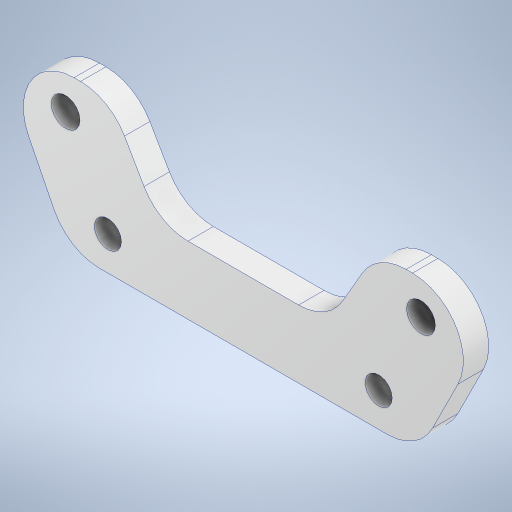
# Autodesk Inventor part: upper_arm
Saved by Autodesk Inventor 2024.1 (Build 281209000, 209)
## iProperties
Created: 2024-02-14
Part Number: upper_arm
Material: アルミニウム 6061
Document SubType Name: Sheet Metal
Designer: hibik
Density: 2.7 g/cm^3
Appearance: アルミニウム - フラット
Sheet Metal Rule: Default
Author: hibik
Autodesk Inventor part; units mm, degrees
ref_plane "YZ Plane" through (0, 0, 0) normal (1, 0, 0) x (0, 1, 0)
ref_plane "XZ Plane" through (0, 0, 0) normal (0, 1, 0) x (-1, 0, 0)
ref_plane "XY Plane" through (0, 0, 0) normal (0, 0, 1) x (1, 0, 0)
sketch "スケッチ2" plane through (0, 0, 0) normal (0, 0, 1) x (1, 0, 0)
  line L0 (0, 0) -> (26, 0)
  line L1 (26, 0) -> (26, 33)
  line L2 (26, 33) -> (0, 33)
  line L3 (0, 33) -> (0, 0)
  line L4 (0, 0) -> (26, 0)
  line L5 (26, 0) -> (26, 24)
  line L6 (26, 24) -> (0, 24) construction
  line L7 (0, 24) -> (0, 0)
  circle A0 centre (13, 24) radius 13
  circle A1 centre (13, 24) radius 6.25
  line L8 (26, 0) -> (0, 0)
  line L9 (0, 0) -> (0, -4)
  line L10 (0, -4) -> (26, -4)
  line L11 (26, -4) -> (26, 0)
  circle A2 centre (21, -2) radius 0.8
  circle A3 centre (5, -2) radius 0.8
  point P0 (22.3808, 33)
  point P1 (3.6192, 33)
  point P2 (26, -2)
  dimension "d0" = 26
  dimension "d1" = 33
  dimension "d2" = 24
  dimension "d3" = 12.5
  dimension "d8" = 4
  dimension "d9" = 1.6
  dimension "d10" = 1.6
  dimension "d12" = 5
  dimension "d13" = 5
  constraints: 24 end point, 6 parallel, 3 centre point, 3 horizontal, 3 perpendicular, 2 horizontal alignment, 2 midpoint, 1 coincident, 1 collinear, 1 point on line, 3 other
  measures "d0" distance of L1.end L2.end
  measures "d1" distance of L2.end L0.start
  measures "d2" distance between parallel lines of L0 L6
  measures "d3" diameter of A1
  measures "d8" distance of L8.end L9.end
  measures "d9" diameter of A2
  measures "d10" diameter of A3
  measures "d12" distance from line of L11 A2.centre
  measures "d13" distance from line of L9 A3.centre
extrude "押し出し1" add sketch "スケッチ2" along normal blind 1.5 contours L3 A0 L1 L0 | L0 L11 L10 L9 | A0 L2 picked at (12.7489, 32.0681)
sketch "スケッチ3" plane through (0, 0, 0) normal (0, 0, -1) x (-1, 0, 0)
  circle A0 centre (-2.5, 24) radius 0.85 projected
  circle A1 centre (-23.5, 24) radius 0.85 projected
  circle A2 centre (-23.5, 3) radius 0.85 projected
  circle A3 centre (-2.5, 3) radius 0.85 projected
  point P0 (0, 0)
extrude "押し出し2" cut sketch "スケッチ3" against normal through all
fillet "フィレット1" radius 3 4 edges at (22.3808, 33, 0.75) (3.6192, 33, 0.75) (26, -4, 0.75) (0, -4, 0.75)
sketch "スケッチ4" plane through (0, 0, 1.5) normal (0, 0, 1) x (1, 0, 0)
  line L0 (0, 24) -> (0, -1) projected
  line L1 (0, 5) -> (26, 5)
  line L2 (26, 5) -> (26, 33)
  line L3 (26, 33) -> (0, 33)
  line L4 (0, 33) -> (0, 5)
  line L5 (21, 33) -> (5, 33) projected
  line L6 (26, -1) -> (26, 24) projected
  circle A0 centre (2.5, 3) radius 0.85 projected
  line L7 (5.1132, 5) -> (8, 0)
  line L8 (8, 0) -> (18, 0)
  line L9 (18, 0) -> (20.8868, 5)
  line L10 (0, 1.2918) -> (2.6459, -4)
  line L11 (3, -4) -> (23, -4) projected
  line L12 (26, 1.2918) -> (23.3541, -4)
  arc A1 (0, -1) -> (3, -4) centre (3, -1) ccw projected
  arc A2 (23, -4) -> (26, -1) centre (23, -1) ccw projected
  line L13 (2.5, 3) -> (5, -2)
  circle A3 centre (5, -2) radius 0.8 projected
  circle A4 centre (21, -2) radius 0.8 projected
  circle A5 centre (23.5, 3) radius 0.85 projected
  line L14 (23.5, 3) -> (21, -2)
  point P0 (0, 0)
  point P1 (13, 0)
  point P2 (13, 5)
  point P3 (23.3653, -3.9777)
  point P4 (2.6347, -3.9777)
  dimension "d15" = 2
  dimension "d16" = 10
  dimension "d17" = 5
  dimension "d18" = 120
  dimension "d19" = 120
  dimension "d24" = 3
  dimension "d25" = 3
  constraints: 22 end point, 7 point on line, 4 parallel, 2 collinear, 2 horizontal, 2 midpoint, 1 coincident, 1 perpendicular, 1 vertical alignment
  measures "d15" distance from line of L1 L13.start
  measures "d16" distance of L7.end L8.end
  measures "d17" distance between parallel lines of L1 L8
  measures "d18" angle of L8 L7
  measures "d19" angle of L9 L8
  measures "d24" distance between parallel lines of L10 L13
  measures "d25" distance between parallel lines of L14 L12
extrude "切り取り1" cut sketch "スケッチ4" against normal blind 3.048 contours L4 L3 L2 L1 L0 | L1 L9 L8 L7
extrude "押し出し3" cut sketch "スケッチ4" against normal through all contours L10 A1 L0 | L6 A2 L12
fillet "フィレット3" radius 3 10 edges at (5.1132, 5, 0.75) (0, 5, 0.75) (8, 0, 0.75) (20.8868, 5, 0.75) (26, 5, 0.75) (26, 1.2918, 0.75) (18, 0, 0.75) (0, 1.2918, 0.75) (2.6347, -3.9777, 0.75) (23.3653, -3.9777, 0.75)
equation "\"d13\" = d12"
equation "\"d19\" = d18"
equation "\"d25\" = d24"
equation "\"d21\" = Thickness"
equation "\"BendRadius\" = Thickness"
equation "\"BendReliefWidth\" = Thickness"
equation "\"BendReliefDepth\" = 0.5 * Thickness"
equation "\"CornerReliefSize\" = 4 * Thickness"
equation "\"MinimumRemnant\" = 2 * Thickness"
equation "\"TransitionRadius\" = BendRadius"
equation "\"JacobiRadiusSize\" = BendRadius"
equation "\"GapSize\" = Thickness"
equation "\"d20\" = Thickness"
equation "\"Thickness\" = 3.048"
